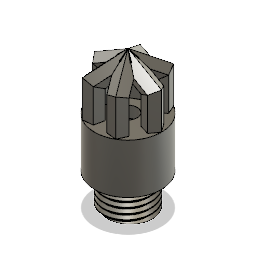
probeTop (Autodesk Fusion 360 design; units mm, degrees)
Autodesk Fusion 360 part; units mm, degrees
note: some values were not read from the file. Chosen so that the rebuilt part matches the saved one: which bodies a step acts on; which face or edge a step refers to; where a thread starts.
sketch "Sketch1" plane through (0, 0, 0) normal (0, 1, 0) x (1, 0, 0)
  circle A0 centre (0, 0) radius 8.75
  dimension "d1" = 17.5
  measures "d1" diameter of A0
extrude "Extrude1" add sketch "Sketch1" along normal blind 21 makes body 1
hole "Hole1" at (-0.0786, 0, -0.0539) direction (0, 1, 0) diameter 4.8 depth 38 tip angle 118 counterbore diameter 8 counterbore depth 18 bodies 1
ref_plane "WorkPlane1" through (0, 8, 0) normal (0, -1, 0) x (-1, 0, 0)
split "Split1" by plane through (0, 8, 0) normal (0, -1, 0) bodies 1 makes body 2 at (8.7065, 5.3333, -0.8712)
thread "Thread1" "ANSI Unified Screw Threads 0.5 1/2-18 UNS 2A" major diameter 12.5578 minor diameter 10.988 pitch 1.4111 angle 60 modelled right hand crest width 0.1764 on face at (8.7065, 5.3333, -0.8712) crest through (6.2789, -0.0882, 0) on bodies 2
sketch "Sketch16" plane through (0, 0, 0) normal (0, 0, 1) x (1, 0, 0)
  line L0 (0, 34.5) -> (-7.7942, 30)
  line L1 (-7.7942, 30) -> (-7.7942, 21)
  line L2 (7.7942, 21) -> (7.7942, 30)
  line L3 (7.7942, 30) -> (0, 34.5)
  line L4 (-2.4786, 21) -> (2.3214, 21)
  point P0 (0, 25.5)
  dimension "d34" = 9
  dimension "d35" = 4.5
  measures "d34" distance of L0.start P0
  measures "d35" distance of P0 L4
ref_plane "WorkPlane6" through (0, 21, 0) normal (0, 1, 0) x (1, 0, 0)
sketch "Sketch17" plane through (0, 21, 0) normal (0, 1, 0) x (1, 0, 0)
  line L0 (-8.75, 0) -> (-7.2126, -2.116)
  line L1 (-7.2126, -2.116) -> (-4.7251, -1.3078)
  line L2 (-4.7251, -1.3078) -> (-4.7251, 1.3078)
  line L3 (-4.7251, 1.3078) -> (-7.2126, 2.116)
  line L4 (-7.2126, 2.116) -> (-8.75, 0)
  point P0 (-6.5251, 0)
  point P1 (-8.75, 0)
  dimension "d45" = 1.8
  measures "d45" distance of P0 L2
sweep "Sweep3" add profiles "Sketch17" path "Sketch16" along L2 L3 L0 L1 section 1 bodies 1
pattern_circular "C-Pattern2" count 3 over 360 about axis through (0, 1.75, 0) along (0, 1, 0) of 20 faces at (8.2375, 27.072, -0.7053) (6.3834, 26.2974, -1.8466) (8.2375, 27.072, 0.7053) (5.3209, 31.9399, -0.7053) (4.7251, 25.8187, -0.4359) (3.9792, 30.5735, -1.8466) (-8.2375, 27.072, 0.7053) (-6.3834, 26.2974, 1.8466) (-4.7251, 25.8187, -0.4359) (-6.3834, 26.2974, -1.8466) (-8.2375, 27.072, -0.7053) (6.3834, 26.2974, 1.8466) (2.9167, 33.328, 0.7053) (-2.9167, 33.328, -0.7053) (1.575, 30.0467, -0.4359) (-2.4042, 31.4829, -1.8466) (-2.9167, 33.328, 0.7053) (-3.9792, 30.5735, 1.8466) (-1.575, 30.0467, -0.4359) (3.9792, 30.5735, 1.8466) on bodies 1
ref_plane "WorkPlane7" through (-8.2806, 27.0476, 2.8274) normal (-0.946356, 0, 0.323126) x (-0.323126, 0, -0.946356)
sketch "Sketch18" plane through (0, 0, 0) normal (0, 1, 0) x (1, 0, 0)
  point P0 (9151051.1364, 92)
combine "Combine1" operation add target body 2 tool bodies 1
